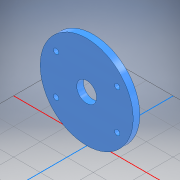
# Autodesk Inventor part: 000.005.005.001 - ОСНОВАНИЕ
Saved by Autodesk Inventor 2022 (Build 260153000, 153)
## iProperties
Created: 2022-12-19
Part Number: 000.005.005.001 - ОСНОВАНИЕ
Material: Пластик АБС
Document SubType Name: Modeling
Designer: Ivan Petrov
Density: 1.06 g/cm^3
Appearance: Голубой
Author: Ivan Petrov
Autodesk Inventor part; units mm, degrees
ref_plane "YZ Plane" through (0, 0, 0) normal (1, 0, 0) x (0, 1, 0)
ref_plane "XZ Plane" through (0, 0, 0) normal (0, 1, 0) x (-1, 0, 0)
ref_plane "XY Plane" through (0, 0, 0) normal (0, 0, 1) x (1, 0, 0)
sketch "Эскиз1" plane through (0, 0, 0) normal (0, 0, 1) x (1, 0, 0)
  circle A0 centre (0, 0) radius 35
  dimension "d7" = 70
  constraints: 1 centre point
  measures "d7" diameter of A0
extrude "Выдавливание1" add sketch "Эскиз1" along normal blind 5
sketch "Эскиз2" plane through (0, 0, 5) normal (0, 0, 1) x (1, 0, 0)
  circle A0 centre (-23, 15) radius 2
  point P0 (0, 0)
  dimension "d4" = 4
  dimension "d5" = 15
  dimension "d6" = 23
  constraints: 1 centre point
  measures "d4" diameter of A0
  measures "d5" vertical distance of A0.centre point (0, 0)
  measures "d6" horizontal distance of point (0, 0) A0.centre
extrude "Выдавливание2" cut sketch "Эскиз2" against normal through all
mirror "Зеркальное отражение1" about plane through (0, 0, 0) normal (0, 1, 0) of "Выдавливание2"
mirror "Зеркальное отражение2" about plane through (0, 0, 0) normal (1, 0, 0) of "Выдавливание2", "Зеркальное отражение1"
sketch "Эскиз19" plane through (0, 0, 5) normal (0, 0, 1) x (1, 0, 0)
  circle A0 centre (0, 0) radius 7.5
  dimension "d75" = 15
  constraints: 1 centre point, 1 coincident
  measures "d75" diameter of A0
extrude "Выдавливание18" cut sketch "Эскиз19" against normal through all
